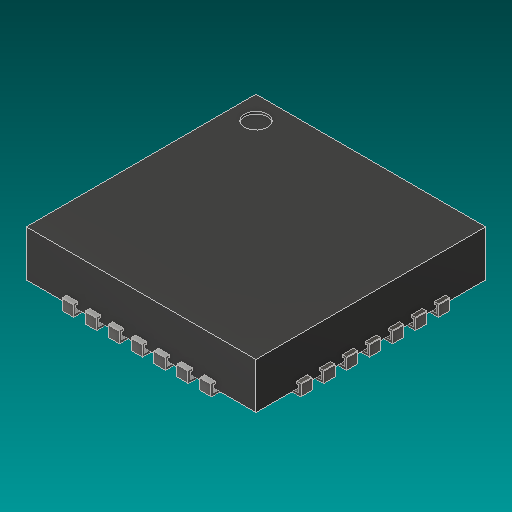
# Autodesk Inventor part: QFN-28
Saved by Autodesk Inventor 2017 (Build 210142000, 142)
## iProperties
Created: 2016-07-01
Part Number: QFN-28
Material: Generic
Document SubType Name: Modeling
Designer: Jonathan
Density: 1 g/cm^3
Appearance: Default
Author: Jonathan
Autodesk Inventor part; units mm, degrees
ref_plane "YZ Plane" through (0, 0, 0) normal (1, 0, 0) x (0, 1, 0)
ref_plane "XZ Plane" through (0, 0, 0) normal (0, 1, 0) x (-1, 0, 0)
ref_plane "XY Plane" through (0, 0, 0) normal (0, 0, 1) x (1, 0, 0)
sketch "Sketch1" plane through (0, 0, 0) normal (0, 1, 0) x (-1, 0, 0)
  line L0 (2.5, 2.5) -> (-2.5, 2.5)
  line L1 (-2.5, 2.5) -> (-2.5, -2.5)
  line L2 (-2.5, -2.5) -> (2.5, -2.5)
  line L3 (2.5, -2.5) -> (2.5, 2.5)
  point P0 (0, 0)
  point P1 (0, -2.5)
  point P2 (2.5, 0)
  dimension "d0" = 5
  dimension "d1" = 5
  constraints: 8 end point, 2 midpoint, 2 parallel, 1 horizontal, 1 horizontal alignment, 1 perpendicular, 1 vertical alignment
  measures "d0" distance of L2.end L0.start
  measures "d1" distance of L1.end L2.end
extrude "Extrusion1" add sketch "Sketch1" along normal blind 1
sketch "Sketch2" plane through (2.5, 0, 2.5) normal (1, 0, 0) x (0, 0, -1)
  line L0 (2.38, 0.15) -> (2.62, 0.15)
  line L1 (2.62, 0.15) -> (2.62, 0.1)
  line L2 (2.62, 0.1) -> (2.38, 0.1)
  line L3 (2.38, 0.1) -> (2.38, 0.15)
  line L4 (0, 0) -> (5, 0) projected
  point P0 (2.5, 0)
  point P1 (2.5, 0.15)
  point P2 (2.5, 0.1)
  point P3 (2.5, 0)
  dimension "d5" = 0.24
  dimension "d6" = 0.05
  dimension "d10" = 0.1
  constraints: 8 end point, 3 midpoint, 2 parallel, 1 horizontal, 1 perpendicular, 1 vertical alignment
  measures "d5" distance of L0.start L0.end
  measures "d6" distance of L2.end L0.start
  measures "d10" distance between parallel lines of L4 L2
extrude "Extrusion2" add sketch "Sketch2" along normal blind 0.1 separate body
sketch "Sketch4" plane through (2.5, 0.1, -0.12) normal (0, -1, 0) x (1, 0, 0)
  line L0 (0.1, 0) -> (0.1, 0.24) projected
  line L1 (0, 0) -> (0.1, 0) projected
  line L2 (0.1, 0.24) -> (0.05, 0.24)
  line L3 (0.05, 0.24) -> (0.05, 0)
  line L4 (0.05, 0) -> (0.1, 0)
  line L5 (0.1, 0) -> (0.1, 0.24)
  point P0 (-2.5, 0.12)
  dimension "d11" = 0.05
  constraints: 8 end point, 2 parallel, 1 horizontal, 1 midpoint, 1 perpendicular
  measures "d11" distance between parallel lines of L3 L0
extrude "Extrusion3" add sketch "Sketch4" along normal blind 0.2 bodies 2
sketch "Sketch7" plane through (2.5, -0.1, -0.12) normal (0, -1, 0) x (1, 0, 0)
  line L0 (0, 0.24) -> (0.1, 0.24) projected
  line L1 (0.05, 0.24) -> (-0.23, 0.24)
  line L2 (0.05, 0.24) -> (0.05, 0) projected
  line L3 (0.05, 0) -> (-0.23, 0)
  arc A0 (-0.23, 0.24) -> (-0.23, 0) centre (-0.23, 0.12) ccw
  line L4 (0.05, 0.24) -> (0.05, 0)
  point P0 (-2.5, 0.12)
  dimension "d19" = 0.28
  constraints: 6 end point, 2 horizontal, 2 point on circle, 2 tangent, 1 centre point, 1 midpoint, 1 perpendicular
  measures "d19" distance of L2.end L3.end
extrude "Extrusion5" add sketch "Sketch7" against normal blind 0.05 bodies 2
fillet "Fillet1" radius 0.01 4 edges at (2.6, -0.1, 0) (2.6, 0.15, 0) (2.55, -0.05, 0) (2.55, 0.1, 0)
pattern_linear "Rectangular Pattern1" count 7 spacing 0.5 along (0, 0, -1) of "Extrusion5", "Fillet1", "Extrusion3", "Extrusion2" first direction both ways yes bodies 2
pattern_circular "Circular Pattern1" count 4 over 360 about axis through (0, -10, 0) along (0, 1, 0) of "Extrusion5", "Fillet1", "Extrusion3", "Extrusion2", "Rectangular Pattern1" bodies 2
sketch "Sketch8" plane through (0, 1, 0) normal (0, 1, 0) x (1, 0, 0)
  circle A0 centre (-2, 2) radius 0.25
  line L0 (2.5, 2.5) -> (-2.5, 2.5) projected
  line L1 (-2.5, 2.5) -> (-2.5, -2.5) projected
  point P0 (0, 0)
  dimension "d29" = 0.5
  dimension "d30" = 0.5
  dimension "d31" = 0.5
  constraints: 1 centre point
  measures "d29" diameter of A0
  measures "d30" distance from line of L0 A0.centre
  measures "d31" distance from line of L1 A0.centre
extrude "Extrusion6" cut sketch "Sketch8" against normal blind 0.05 bodies 1
sketch "Sketch9" plane through (0, 0, 0) normal (0, -1, 0) x (1, 0, 0)
  line L0 (-1.05, 1.05) -> (1.05, 1.05)
  line L1 (1.05, 1.05) -> (1.05, -1.05)
  line L2 (1.05, -1.05) -> (-0.6964, -1.05)
  line L3 (-1.05, -0.6964) -> (-1.05, 1.05)
  line L4 (-1.05, -0.6964) -> (-0.6964, -1.05)
  point P0 (0, 0)
  point P1 (0, 1.05)
  point P2 (1.05, 0)
  dimension "d34" = 2.1
  dimension "d35" = 0.5
  constraints: 10 end point, 3 perpendicular, 2 midpoint, 2 parallel, 1 horizontal, 1 horizontal alignment, 1 vertical alignment
  measures "d34" distance of L0.end L1.end
  measures "d35" distance of L3.start L2.end
extrude "Extrusion7" add sketch "Sketch9" along normal blind 0.05 separate body
body "Solid1"
body "Solid2"
body "Solid3"
